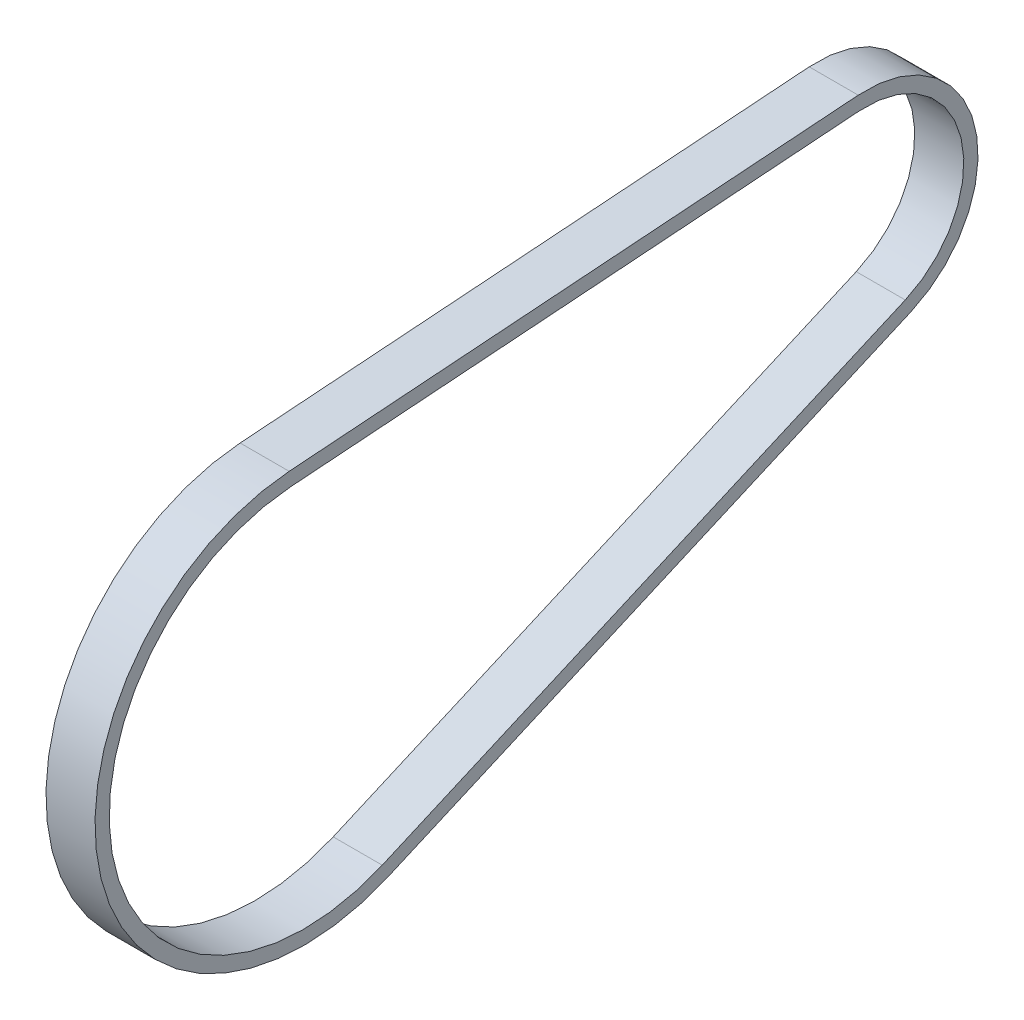
# Autodesk Inventor part: ChassiBelt4.0
Saved by Autodesk Inventor 2023 (Build 270158000, 158)
## iProperties
Created: 2022-10-05
Part Number: ChassiBelt4.0
Material: Generic
Document SubType Name: Modeling
Designer: deli
Density: 1 g/cm^3
Appearance: Default
Author: deli
Autodesk Inventor part; units mm, degrees
ref_plane "YZ Plane" through (0, 0, 0) normal (1, 0, 0) x (0, 1, 0)
ref_plane "XZ Plane" through (0, 0, 0) normal (0, 1, 0) x (-1, 0, 0)
ref_plane "XY Plane" through (0, 0, 0) normal (0, 0, 1) x (1, 0, 0)
sketch "Sketch1" plane through (0, 0, 0) normal (1, 0, 0) x (0, 1, 0)
  circle A0 centre (73.477, -61.6398) radius 2 construction
  circle A1 centre (56.527, 7.1292) radius 2 construction
  arc A2 (62.5344, -66.4088) -> (85.3824, -60.7773) centre (73.477, -61.6398) ccw
  arc A3 (80.3378, 8.8542) -> (34.6419, -2.4088) centre (56.527, 7.1292) ccw
  line L0 (85.3824, -60.7773) -> (80.3378, 8.8542)
  line L1 (62.5344, -66.4088) -> (34.6419, -2.4088)
  line L2 (82.0733, 8.98) -> (87.1179, -60.6516)
  arc A4 (60.9394, -67.104) -> (87.1179, -60.6516) centre (73.477, -61.6398) ccw
  line L3 (60.9394, -67.104) -> (33.0468, -3.104)
  arc A5 (82.0733, 8.98) -> (33.0468, -3.104) centre (56.527, 7.1292) ccw
  point P0 (0, 0)
  dimension "d0" = 23.8732
  dimension "d1" = 47.7465
  dimension "d2" = 1.74
  constraints: 8 end point, 8 point on circle, 4 centre point, 4 tangent, 2 coincident, 3 other
  measures "d0" diameter of A2
  measures "d1" diameter of A3
  measures "d2" distance between parallel lines of L0 L2
extrude "Extrusion1" add sketch "Sketch1" along normal blind 6
body "Solid1"
